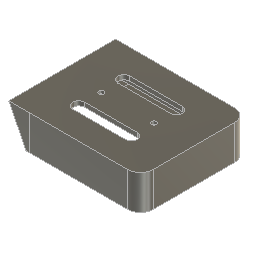
Крепление аккамулятора Milwaukee_ver4 (Autodesk Fusion 360 design; units mm, degrees)
Autodesk Fusion 360 part; units mm, degrees
note: some values were not read from the file. Set by a fixed rule: which sketch regions a step uses.
sketch "Sketch1" plane through (0, 0, 0) normal (0, 0, 1) x (1, 0, 0)
  line L0 (36.5, 30.5) -> (-32.5, 30.5)
  line L1 (-32.5, 30.5) -> (-32.5, -30.5)
  line L2 (-32.5, -30.5) -> (36.5, -30.5)
  line L3 (36.5, -30.5) -> (36.5, 30.5)
  line L4 (36.5, -27.25) -> (-32.5, -27.25)
  line L5 (-32.5, -27.25) -> (-32.5, 27.25)
  line L6 (-32.5, 27.25) -> (36.5, 27.25)
  line L7 (36.5, 27.25) -> (36.5, -27.25)
  line L8 (33, 35.5) -> (-32.5, 35.5)
  line L9 (-32.5, 35.5) -> (-32.5, 30.5)
  line L10 (1.75, 0) -> (22.5, 0)
  line L11 (-32.5, -35.5) -> (-32.5, -30.5)
  line L12 (32.9935, -35.55) -> (-32.5, -35.5)
  line L13 (41.5, -27.05) -> (41.5, 27)
  arc A0 (32.9935, -35.55) -> (41.5, -27.05) centre (33, -27.05) ccw
  arc A1 (41.5, 27) -> (33, 35.5) centre (33, 27) ccw
  dimension "d1" = 69
  dimension "d2" = 61
  dimension "d3" = 69
  dimension "d4" = 54.5
  dimension "d46" = 8.5
  constraint horizontal L0
  constraint perpendicular L0 L1
  constraint parallel L0 L2
  constraint parallel L1 L3
  constraint horizontal L4
  constraint perpendicular L4 L5
  constraint parallel L4 L6
  constraint parallel L5 L7
  constraint perpendicular L0 L9
  constraint symmetric L0.end L10 L1.end
  constraint symmetric L8.end L10 L11.start
  constraint tangent L13 A0
  constraint tangent L12 A0
  constraint tangent L8 A1
  constraint tangent L13 A1
  constraint equal A0 A1
  measures "d1" distance of L1.end L2.end
  measures "d2" distance of L0.end L1.end
  measures "d3" distance of L5.end L6.end
  measures "d4" distance of L4.end L5.end
  measures "d46" radius of A0
extrude "Extrude1" add sketch "Sketch1" along normal blind 6.45 contours L0 L1 L3 L6 | L0 L2 L3 L7 L8 L9 L11 L12 L13 A0 A1 | L1 L2 L3 L4
extrude "Extrude2" add sketch "Sketch1" along normal blind 22 contours L0 L2 L3 L7 L8 L9 L11 L12 L13 A0 A1
extrude "Extrude3" add sketch "Sketch1" along normal blind 23 and the other way blind -20
sketch "Sketch2" plane through (0, 0, 23) normal (0, 0, 1) x (-1, 0, 0)
  line L0 (-33, -35.5) -> (32.5, -35.5)
  line L1 (32.5, -35.5) -> (32.5, 35.5)
  line L2 (32.5, 35.5) -> (-32.9935, 35.55)
  circle A0 centre (20, 0) radius 1.75
  circle A1 centre (-15, 0) radius 1.75
  arc A2 (-32.9935, 35.55) -> (-41.5, 27.05) centre (-33, 27.05) ccw
  line L3 (-41.5, 27.05) -> (-41.5, -27)
  arc A3 (-41.5, -27) -> (-33, -35.5) centre (-33, -27) ccw
  dimension "d33" = 3.5
  dimension "d34" = 3.5
  measures "d33" diameter of A0
  measures "d34" diameter of A1
extrude "Extrude4" cut sketch "Sketch2" against normal blind 5 contours A0 | A1
sketch "Sketch3" plane through (0, 35.5, 0) normal (0, 1, 0) x (-1, 0, 0)
  line L0 (-33, 0) -> (32.5, 0)
  line L1 (32.5, 0) -> (32.5, 23)
  line L2 (32.5, 23) -> (-33, 23)
  line L3 (32.5, 23) -> (34.5, 23)
  line L4 (34.5, 23) -> (34.5, 0)
  line L5 (34.5, 0) -> (32.5, 0)
  line L6 (34.5, 0) -> (34.5, 8)
  line L7 (34.5, 23) -> (46.0025, 23)
  line L8 (34.5, 0) -> (46.0025, 23)
  line L9 (-33, 23) -> (-33, 0)
  dimension "d47" = 26.57
  constraint coincident L1.end L2.start
  constraint perpendicular L1 L3
  constraint perpendicular L3 L4
  constraint coincident L0.end L1.start
  constraint perpendicular L1 L5
  constraint coincident L4 L6.end
  constraint perpendicular L4 L7
  measures "d47" angle of L4 L8
extrude "Extrude5" add sketch "Sketch3" against normal blind 5 contours L1 L3 L4 L5 L6 | L4 L6 L7 L8
extrude "Extrude6" add sketch "Sketch3" along normal blind -71 and the other way blind 66 contours L1 L3 L4 L5 L6 | L4 L6 L7 L8
sketch "Sketch4" plane through (0, 30.5, 0) normal (0, -1, 0) x (1, 0, 0)
  line L0 (-32.5, 20) -> (-32.5, 23)
  line L1 (-32.5, 23) -> (-46.0025, 23)
  line L2 (-46.0025, 23) -> (-34.5, 0)
  line L3 (-34.5, 0) -> (-37.7235, 6.4455)
  line L4 (-32.5, 6.4455) -> (-37.7235, 6.4455)
  line L5 (-32.5, 6.4455) -> (-32.5, 0)
  line L6 (-34.5, 0) -> (-32.5, 0)
  line L7 (36.5, 20) -> (-32.5, 20)
  line L8 (-32.5, 6.45) -> (36.5, 6.45)
  line L9 (36.5, 6.45) -> (36.5, 20)
  constraint coincident L2.end L3.start
  constraint perpendicular L4 L5
  constraint perpendicular L5 L6
  constraint coincident L2 L3.end
extrude "Extrude7" add sketch "Sketch4" along normal blind 3.25
extrude "Extrude8" add sketch "Sketch4" along normal blind 61 and the other way blind -57.75
chamfer "Chamfer2" distance 1 angle 45 2 edges at (-18.3684, 0.6328, 20) (16.6316, 0.6328, 20)
sketch "Sketch5" plane through (0, 30.5, 0) normal (0, -1, 0) x (1, 0, 0)
  line L0 (-37.7235, 6.4455) -> (-32.5, 6.4455)
  line L1 (-32.5, 6.4455) -> (-32.5, 6.45)
  line L2 (-46.0025, 23) -> (-37.7235, 6.4455)
  line L3 (-32.5, 6.45) -> (36.5, 6.45)
  line L4 (36.5, 6.45) -> (36.5, 20)
  line L5 (36.5, 20) -> (-32.5, 20)
  line L6 (-46.0025, 23) -> (-27, 23)
  line L7 (-29, 20) -> (-51.5326, 20)
  line L8 (-43.3815, 17.7592) -> (-46.4301, 23.8551)
  line L9 (-28, 19) -> (-27.5232, 25.3132)
  constraint coincident L2.start L6.start
  constraint horizontal L6
  constraint coincident L5 L7.start
  constraint coincident L2 L8.start
  constraint parallel L2 L8
extrude "Extrude9" add sketch "Sketch5" along normal blind 61 contours L2 L5 L6 L7 L8 L9
sketch "Sketch6" plane through (0, 0, 20) normal (0, 0, -1) x (1, 0, 0)
  circle A0 centre (-20, 0) radius 2.75
  line L0 (36.5, 30.5) -> (-44.5022, 30.5)
  line L1 (-44.5022, -30.5) -> (36.5, -30.5)
  line L2 (36.5, -30.5) -> (36.5, 30.5)
  circle A1 centre (15, 0) radius 2.75
  line L3 (15, -11) -> (-20, -11)
  arc A2 (-20, -11) -> (-20, -19) centre (-20, -15) ccw
  line L4 (-20, -19) -> (15, -19)
  arc A3 (15, -19) -> (15, -11) centre (15, -15) ccw
  line L5 (15, -15) -> (-20, -15) construction
  line L6 (1.75, 0) -> (22.5, 0)
  line L7 (-20, 19) -> (15, 19)
  arc A4 (15, 11) -> (15, 19) centre (15, 15) ccw
  line L8 (15, 11) -> (-20, 11)
  arc A5 (-20, 19) -> (-20, 11) centre (-20, 15) ccw
  line L9 (-44.5022, 30.5) -> (-44.5022, -30.5)
  constraint tangent L3 A2
  constraint tangent A2 L4
  constraint parallel L3 L4
  constraint tangent L4 A3
  constraint tangent L3 A3
  constraint horizontal L5
  constraint symmetric L3.start L6 A4.start
  constraint symmetric L3.end L6 L8.end
  constraint symmetric A2.end L6 L7.start
  constraint symmetric L4.end L6 L7.end
  constraint symmetric A2 L6 A5
  constraint symmetric A3 L6 A4
extrude "Extrude10" cut sketch "Sketch6" against normal blind 25 contours L3 A2 L4 A3 | L7 A4 L8 A5
